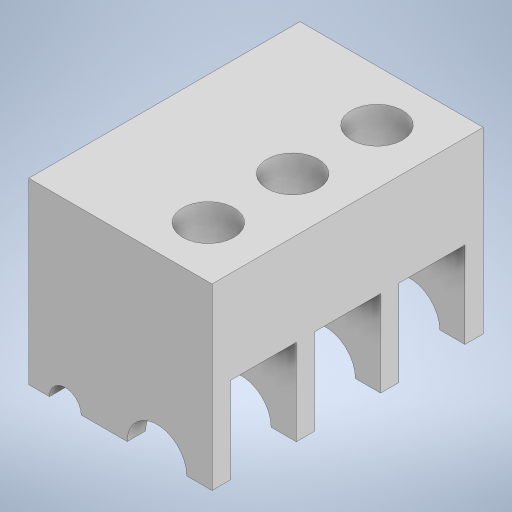
# Autodesk Inventor part: E.Engine Block Bottom
Saved by Autodesk Inventor 2023 (Build 270158000, 158)
## iProperties
Created: 2023-01-04
Part Number: E.Engine Block Bottom
Material: Generic
Document SubType Name: Modeling
Designer: tgr41
Density: 1 g/cm^3
Appearance: Default
Mass: 1928.08 g
Surface Area: 1645.68 cm^2
Volume: 1928.08 cm^3
Author: tgr41
Autodesk Inventor part; units mm, degrees
ref_plane "YZ Plane" through (0, 0, 0) normal (1, 0, 0) x (0, 1, 0)
ref_plane "XZ Plane" through (0, 0, 0) normal (0, 1, 0) x (-1, 0, 0)
ref_plane "XY Plane" through (0, 0, 0) normal (0, 0, 1) x (1, 0, 0)
sketch "Sketch1" plane through (0, 0, 0) normal (0, 0, 1) x (1, 0, 0)
  line L0 (127, 0) -> (127, 123.9012)
  line L1 (127, 123.9012) -> (0, 123.9012)
  line L2 (0, 123.9012) -> (0, 0)
  arc A0 (109.5375, 0) -> (68.2625, 0) centre (88.9, 0) ccw
  arc A1 (36.3964, 0) -> (14.4, 0) centre (25.3982, 0) ccw
  line L3 (14.4, 0) -> (0, 0)
  line L4 (127, 0) -> (109.5375, 0)
  line L5 (68.2625, 0) -> (36.3964, 0)
  dimension "d0" = 127
  dimension "d1" = 123.9012
  dimension "d2" = 41.275
  dimension "d25" = 38.1
  dimension "d26" = 21.9964
  constraints: 12 end point, 4 point on circle, 3 horizontal, 2 centre point, 1 parallel
  measures "d0" distance of L1.end L0.end
  measures "d1" distance of L0.end L0.start
  measures "d2" diameter of A0
  measures "d25" distance from line of L0 A0.centre
  measures "d26" diameter of A1
extrude "Extrusion1" add sketch "Sketch1" along normal blind 187.96
sketch "Sketch2" plane through (0, 123.9012, 0) normal (0, 1, 0) x (1, 0, 0)
  circle A0 centre (88.9, -152.4) radius 17.78
  line L0 (127, -187.96) -> (0, -187.96) projected
  line L1 (127, 0) -> (127, -187.96) projected
  circle A1 centre (88.9, -93.98) radius 17.78
  circle A2 centre (88.9, -35.56) radius 17.78
  line L2 (127, 0) -> (0, 0) projected
  point P0 (127, -35.56)
  point P1 (127, -93.98)
  point P2 (127, -152.4)
  dimension "d6" = 35.56
  dimension "d7" = 38.1
  dimension "d10" = 35.56
  dimension "d11" = 38.1
  dimension "d13" = 58.42
  dimension "d14" = 38.1
  dimension "d29" = 35.56
  constraints: 3 centre point, 2 equal radius, 2 point on line, 1 midpoint
  measures "d6" distance from line of L0 A0.centre
  measures "d7" distance from line of L1 A0.centre
  measures "d10" distance from line of L2 A2.centre
  measures "d11" distance from line of L1 A2.centre
  measures "d13" distance of A1.centre A0.centre
  measures "d14" distance from line of L1 A1.centre
  measures "d29" diameter of A2
sketch "Sketch3" plane through (127, 0, 0) normal (1, 0, 0) x (0, 0, -1)
  line L0 (0, 123.9012) -> (-187.96, 123.9012) projected
  line L1 (0, 0) -> (-187.96, 0) projected
  line L2 (-35.56, 59.69) -> (-35.56, 0)
  line L3 (0, 0) -> (-187.96, 0) projected
  line L4 (-93.98, 0) -> (-93.98, 59.69)
  line L5 (-152.4, 59.69) -> (-152.4, 0)
  line L6 (0, 0) -> (0, 123.9012) projected
  line L7 (-187.96, 0) -> (-175.26, 0)
  line L8 (-175.26, 0) -> (-175.26, 59.69)
  line L9 (-175.26, 123.9012) -> (-187.96, 123.9012)
  line L10 (-187.96, 123.9012) -> (-187.96, 0)
  line L11 (-116.84, 0) -> (-129.54, 0)
  line L12 (-129.54, 0) -> (-129.54, 59.69)
  line L13 (-129.54, 123.9012) -> (-116.84, 123.9012)
  line L14 (-116.84, 59.69) -> (-116.84, 0)
  line L15 (-35.56, 59.69) -> (-35.56, 0)
  line L16 (0, 0) -> (-12.7, 0)
  line L17 (-12.7, 0) -> (-12.7, 59.69)
  line L18 (-12.7, 123.9012) -> (0, 123.9012)
  line L19 (0, 123.9012) -> (0, 0)
  line L20 (-71.12, 0) -> (-58.42, 0)
  line L21 (-58.42, 0) -> (-58.42, 59.69)
  line L22 (-58.42, 123.9012) -> (-71.12, 123.9012)
  line L23 (-71.12, 59.69) -> (-71.12, 0)
  line L24 (-187.96, 123.9012) -> (-187.96, 0) projected
  line L25 (-187.96, 123.9012) -> (0, 123.9012)
  line L26 (-58.42, 59.69) -> (-12.7, 59.69)
  line L27 (-175.26, 59.69) -> (-129.54, 59.69)
  line L28 (-116.84, 59.69) -> (-71.12, 59.69)
  dimension "d15" = 35.56
  dimension "d16" = 93.98
  dimension "d17" = 152.4
  dimension "d18" = 12.7
  constraints: 48 end point, 14 symmetric about line, 7 perpendicular, 4 midpoint, 3 point on line, 2 horizontal, 2 parallel
  measures "d15" distance between parallel lines of L6 L2
  measures "d16" distance between parallel lines of L6 L4
  measures "d17" distance between parallel lines of L6 L5
  measures "d18" distance of L9.end L9.start
extrude "Extrusion2" cut sketch "Sketch3" against normal blind 187.96 contours L1 L2 L26 L17 | L1 L21 L26 L2 | L1 L4 L28 L23 | L1 L14 L28 L4 | L1 L5 L27 L12 | L8 L27 L5 L1
extrude "Extrusion3" cut sketch "Sketch2" against normal blind 187.96
sketch "Sketch4" plane through (127, 59.69, 129.54) normal (0, -1, 0) x (1, 0, 0)
  line L0 (-58.7375, -116.84) -> (-90.6036, -116.84) projected
  line L1 (-74.6705, -116.84) -> (-74.6705, 45.72)
  line L2 (-90.6036, 45.72) -> (-58.7375, 45.72) projected
  line L3 (-74.6705, 45.72) -> (-127, 45.72)
  line L4 (-127, -116.84) -> (-127, -71.12) projected
  line L5 (-127, 45.72) -> (-127, -116.84)
  line L6 (-127, -116.84) -> (-74.6705, -116.84)
  point P0 (-127, -129.54)
  constraints: 8 end point, 2 midpoint, 1 collinear, 1 horizontal, 1 perpendicular
extrude "Extrusion4" add sketch "Sketch4" along normal blind 38.1
body "Solid1"
